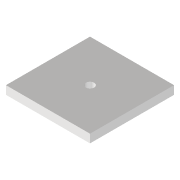
# Autodesk Inventor part: 00_mirror_tmp
Saved by Autodesk Inventor 2022 (Build 260153000, 153)
## iProperties
Created: 2023-01-02
Part Number: 00_mirror_tmp
Material: Generisch
Document SubType Name: Modeling
Designer: diederichbenedict
Density: 1 g/cm^3
Appearance: Vorgabe
Author: diederichbenedict
Autodesk Inventor part; units mm, degrees
ref_plane "YZ Plane" through (0, 0, 0) normal (1, 0, 0) x (0, 1, 0)
ref_plane "XZ Plane" through (0, 0, 0) normal (0, 1, 0) x (-1, 0, 0)
ref_plane "XY Plane" through (0, 0, 0) normal (0, 0, 1) x (1, 0, 0)
sketch "Skizze1" plane through (0, 0, 0) normal (0, 1, 0) x (-1, 0, 0)
  line L0 (-5, -5) -> (5, -5)
  line L1 (5, -5) -> (5, 5)
  line L2 (5, 5) -> (-5, 5)
  line L3 (-5, 5) -> (-5, -5)
  line L4 (-5, -5) -> (5, 5) construction
  line L5 (5, -5) -> (-5, 5) construction
  circle A0 centre (0, 0) radius 0.5
  dimension "d0" = 10
  dimension "d1" = 10
  dimension "d4" = 1
  constraints: 12 end point, 2 midpoint, 2 parallel, 1 centre point, 1 coincident, 1 horizontal, 1 perpendicular
  measures "d0" distance of L2.end L1.end
  measures "d1" distance of L1.end L0.end
  measures "d4" diameter of A0
extrude "Extrusion1" add sketch "Skizze1" along normal blind 1
equation "\"d1\" = d0"
